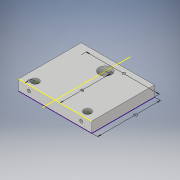
# Autodesk Inventor part: ABI_Grundplatte
Saved by Autodesk Inventor 2018.3 (Build 223284000, 284)
## iProperties
Created: 2019-11-22
Part Number: ABI_Grundplatte
Material: Generisch
Document SubType Name: Modeling
Designer: maascl
Density: 1 g/cm^3
Appearance: Vorgabe
Author: maascl
Autodesk Inventor part; units mm, degrees
ref_plane "YZ Plane" through (0, 0, 0) normal (1, 0, 0) x (0, 1, 0)
ref_plane "XZ Plane" through (0, 0, 0) normal (0, 1, 0) x (-1, 0, 0)
ref_plane "XY Plane" through (0, 0, 0) normal (0, 0, 1) x (1, 0, 0)
sketch "Skizze1" plane through (0, 0, 0) normal (0, 0, 1) x (1, 0, 0)
  line L0 (-35, -30) -> (35, -30)
  line L1 (35, -30) -> (35, 30)
  line L2 (35, 30) -> (-35, 30)
  line L3 (-35, 30) -> (-35, -30)
  line L4 (-35, -30) -> (35, 30) construction
  line L5 (35, -30) -> (-35, 30) construction
  point P0 (0, 0)
  dimension "Breite" = 70
  dimension "Länge" = 60
  constraints: 12 end point, 2 midpoint, 2 parallel, 1 horizontal, 1 perpendicular
  measures "Breite" distance between parallel lines of L1 L3
  measures "Länge" distance between parallel lines of L2 L0
extrude "Extrusion1" add sketch "Skizze1" along normal blind 10
sketch "Skizze2" plane through (0, 0, 10) normal (0, 0, 1) x (1, 0, 0)
  line L0 (-35, -30) -> (35, -30) projected
  line L1 (0, -42) -> (0, 42) projected
  point P0 (0, 0)
  point P1 (-25, -24)
  point P2 (25, -24)
  point P3 (0, 18)
  dimension "Abstand_bohrung_unten" = 6
  dimension "Abstand_Bohrung_oben" = 48
  constraints: 1 symmetric about line
  measures "Abstand_bohrung_unten" distance from line of L0 point (-25, -24)
  measures "Abstand_Bohrung_oben" distance from line of L0 point (0, 18)
hole "Bohrung1" at (25, -24, 10) at (-25, -24, 10) direction (0, 0, -1) diameter 7 end through all
hole "Bohrung2" at (0, 18, 10) direction (0, 0, -1) diameter 12 end through all
sketch "Skizze3" plane through (-35, -30, 0) normal (0, -1, 0) x (1, 0, 0)
  line L0 (35, -2) -> (35, 12) projected
  point P0 (35, 0)
  point P1 (10, 5)
  point P2 (60, 5)
  dimension "Abstand_Seitenlöcher_unten" = 50
  constraints: 1 symmetric about line
  measures "Abstand_Seitenlöcher_unten" distance of point (60, 5) point (10, 5)
hole "Bohrung3" at (-25, -30, 5) at (25, -30, 5) direction (0, 1, 0) diameter 3 depth 15 tip angle 118
sketch "Skizze4" plane through (-35, 30, 0) normal (0, 1, 0) x (1, 0, 0)
  line L0 (0, 0) -> (0, -10) projected
  point P0 (35, 0)
  point P1 (35, -5)
  dimension "Abstand_Bohrung_Seitenlöcher_oben" = 35
  measures "Abstand_Bohrung_Seitenlöcher_oben" distance from line of L0 point (35, -5)
hole "Bohrung4" at (0, 30, 5) direction (0, -1, 0) diameter 3 depth 15 tip angle 118
